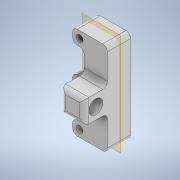
# Autodesk Inventor part: STUURAS
Saved by Autodesk Inventor 2022 (Build 260153000, 153)
## iProperties
Created: 2021-12-21
Part Number: STUURAS
Material: Generic
Document SubType Name: Modeling
Designer: keemi
Density: 1 g/cm^3
Appearance: Default
Author: keemi
Autodesk Inventor part; units mm, degrees
ref_plane "YZ Plane" through (0, 0, 0) normal (1, 0, 0) x (0, 1, 0)
ref_plane "XZ Plane" through (0, 0, 0) normal (0, 1, 0) x (-1, 0, 0)
sketch "Sketch1" plane through (0, 0, 0) normal (0, 1, 0) x (-1, 0, 0)
  line L0 (0, 0) -> (10, 0)
  line L1 (10, 0) -> (10, -10)
  line L2 (10, -10) -> (0, -10)
  line L3 (0, -10) -> (0, 0)
  dimension "d0" = 10
  dimension "d1" = 10
  constraints: 8 end point, 2 parallel, 1 horizontal, 1 perpendicular
  measures "d0" distance of L1.end L2.end
  measures "d1" distance of L0.end L1.end
extrude "Extrusion1" add sketch "Sketch1" along normal blind 40
sketch "Sketch2" plane through (-10, 0, -10) normal (-1, 0, 0) x (0, 0, 1)
  line L0 (0, 40) -> (10, 40) projected
  line L1 (10, 40) -> (0, 40)
  line L2 (0, 40) -> (0, 34)
  line L3 (0, 34) -> (10, 34)
  line L4 (10, 34) -> (10, 40)
  point P0 (10, 0)
  dimension "d4" = 10
  dimension "d5" = 6
  constraints: 8 end point, 2 parallel, 1 horizontal, 1 perpendicular
  measures "d4" distance of L3.end L2.end
  measures "d5" distance of L2.end L1.end
extrude "Extrusion2" add sketch "Sketch2" along normal blind 5
sketch "Sketch3" plane through (-10, 0, -10) normal (-1, 0, 0) x (0, 0, 1)
  line L0 (10, 0) -> (10, 40) projected
  line L1 (10, 0) -> (0, 0)
  line L2 (0, 0) -> (0, 6)
  line L3 (0, 6) -> (10, 6)
  line L4 (10, 6) -> (10, 0)
  dimension "d8" = 10
  dimension "d9" = 6
  constraints: 8 end point, 2 parallel, 1 horizontal, 1 perpendicular
  measures "d8" distance of L2.end L3.end
  measures "d9" distance of L1.end L2.end
extrude "Extrusion3" add sketch "Sketch3" along normal blind 5
sketch "Sketch4" plane through (-10, 34, -10) normal (-1, 0, 0) x (0, 0, 1)
  line L0 (10, -34) -> (10, 6) projected
  line L1 (10, -34) -> (10, -14)
  line L2 (10, -14) -> (10, -17)
  line L3 (10, -17) -> (0, -17)
  line L4 (0, -17) -> (0, -11)
  line L5 (0, -11) -> (10, -11)
  line L6 (10, -11) -> (10, -17)
  point P0 (10, -11)
  dimension "d12" = 20
  dimension "d13" = 3
  dimension "d14" = 10
  dimension "d15" = 6
  constraints: 12 end point, 2 parallel, 1 horizontal, 1 midpoint, 1 perpendicular, 1 point on line
  measures "d12" distance of L0.start L1.end
  measures "d13" distance of L1.end L2.end
  measures "d14" distance of L4.end L5.end
  measures "d15" distance of L3.end L4.end
extrude "Extrusion4" add sketch "Sketch4" along normal blind 5
sketch "Sketch5" plane through (0, 0, 0) normal (0, 0, 1) x (1, 0, 0)
  line L0 (-15, 0) -> (-15, 6) projected
  line L1 (-15, 3) -> (-12, 3)
  line L2 (-15, 23) -> (-15, 17) projected
  line L3 (-15, 20) -> (-12, 20)
  line L4 (-15, 34) -> (-15, 40) projected
  line L5 (-15, 37) -> (-12, 37)
  point P0 (0, 0)
  dimension "d18" = 3
  dimension "d19" = 3
  dimension "d20" = 3
  constraints: 6 end point, 3 horizontal, 3 midpoint
  measures "d18" distance of L1.start L1.end
  measures "d19" distance of L3.start L3.end
  measures "d20" distance of L5.start L5.end
hole "Hole1" at (-12, 37, 0) at (-12, 20, 0) at (-12, 3, 0) direction (0, 0, -1) diameter 3 end through all
fillet "Fillet1" radius 2 8 edges at (-15, 17, -5) (-15, 23, -5) (-15, 40, -5) (-15, 34, -5) (-15, 6, -5) (-15, 0, -5) (0, 40, -5) (0, 0, -5)
sketch "Sketch6" plane through (0, 2, -10) normal (1, 0, 0) x (0, 0, -1)
  point P0 (-10, -2)
sketch "Sketch7" plane through (0, 0, 0) normal (0, 0, 1) x (1, 0, 0)
  point P0 (0, 0)
ref_plane "Work Plane1" through (0, 0, -5) normal (0, 0, 1) x (1, 0, 0)
sketch "Sketch10" plane through (0, 0, -5) normal (0, 0, 1) x (1, 0, 0)
  point P0 (0, 0)
sketch "Sketch12" plane through (-10, 23, 0) normal (0, 0, 1) x (1, 0, 0)
  line L0 (10, -23) -> (10, -3)
  line L1 (10, -23) -> (30, -23) construction
  line L2 (10, -3) -> (10, 2)
  line L3 (0, 0) -> (0, 11) projected
  line L4 (10, 2) -> (0, 2)
  line L5 (0, 2) -> (0, -8)
  line L6 (0, -8) -> (10, -8)
  line L7 (10, -8) -> (10, 2)
  dimension "d45" = 20
  dimension "d46" = 90
  dimension "d47" = 5
  dimension "d48" = 10
  dimension "d49" = 10
  constraints: 14 end point, 3 parallel, 2 horizontal, 2 perpendicular, 1 vertical
  measures "d45" distance of L0.start L0.end
  measures "d46" angle of L1 L0
  measures "d47" distance of L0.end L2.end
  measures "d48" distance of L6.end L5.end
  measures "d49" distance of L5.end L4.end
extrude "Extrusion6" add sketch "Sketch12" along normal blind 10
fillet "Fillet2" radius 2 9 edges at (-5, 15, 0) (-5, 15, 10) (-5, 25, 10) (-5, 25, 0) (0, 20, 10) (-10, 20, 10) (-10, 23, -5) (-10, 34, -5) (-10, 6, -5)
fillet "Fillet3" radius 2 1 edges at (-10, 17, -5)
sketch "Sketch13" plane through (0, 2, -10) normal (1, 0, 0) x (0, 0, -1)
  line L0 (-12, 13) -> (-18, 13) projected
  line L1 (-18, 13) -> (-18, 18)
  line L2 (-18, 23) -> (-18, 13) projected
  line L3 (-18, 18) -> (-15, 18)
  circle A0 centre (-15, 18) radius 3
  point P0 (-10, -2)
  dimension "d54" = 5
  dimension "d55" = 3
  dimension "d56" = 6
  constraints: 4 end point, 1 centre point, 1 coincident, 1 midpoint, 1 perpendicular
  measures "d54" distance of L0.end L1.end
  measures "d55" distance of L1.end L3.end
  measures "d56" diameter of A0
extrude "Extrusion7" cut sketch "Sketch13" against normal blind 10
body "Solid1"
